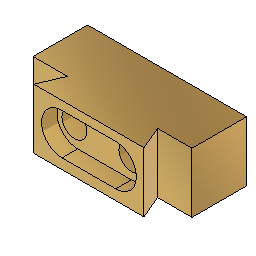
Low Profile Vice Base v5 (Autodesk Fusion 360 archive; units mm, degrees)
design "Vice Piece Hex Only"
Autodesk Fusion 360 part; units mm, degrees
sketch "Sketch1" plane through (0, 0, 0) normal (0, 0, 1) x (1, 0, 0)
  line L0 (-13.9084, 7.56) -> (36.9716, 7.56)
  line L1 (36.9716, 7.56) -> (36.9716, 25.03)
  line L2 (36.9716, 25.03) -> (-13.9084, 25.03)
  line L3 (-13.9084, 25.03) -> (-13.9084, 7.56)
  line L4 (-13.9084, 7.56) -> (-2.9084, 7.56) construction
  line L5 (36.9716, 7.56) -> (25.9716, 7.56) construction
  dimension "d4" = 50.88
  dimension "d5" = 17.47
  dimension "d7" = 11
  dimension "d8" = 11
  constraint horizontal L0
  constraint vertical L1
  constraint horizontal L2
  constraint vertical L3
  constraint perpendicular L3 L4
  constraint perpendicular L1 L5
  measures "d4" distance of L0.start L0.end
  measures "d5" distance of L0.start L2.end
  measures "d7" distance of L0.start L4.end
  measures "d8" distance of L0.end L5.end
sketch "Sketch2" plane through (0, 0, 0) normal (0, 0, 1) x (1, 0, 0)
  line L0 (11.5316, 0) -> (29.1316, 0)
  line L1 (11.5316, 0) -> (-6.0684, 0)
  line L2 (-13.9084, 7.56) -> (36.9716, 7.56)
  line L3 (-2.9084, 7.56) -> (-6.0684, 0)
  line L4 (25.9716, 7.56) -> (29.1316, 0)
  point P0 (-2.9084, 7.56)
  point P1 (25.9716, 7.56)
  dimension "d9" = 17.6
  dimension "d10" = 17.6
  dimension "d11" = 7.56
  constraint coincident P0 L3.start
  constraint coincident P1 L4.start
  measures "d9" distance of L0.start L0.end
  measures "d10" distance of L0.start L1.end
  measures "d11" distance of L0 L2
extrude "Extrude1" add sketch "Sketch1" sketch "Sketch2" along normal blind 19.16 of sketch 2
sketch "Sketch4" plane through (0, 0, 0) normal (0, 1, 0) x (1, 0, 0)
  circle A0 centre (2.9316, -9.8352) radius 6.57
  line L0 (-6.0684, 0) -> (-6.0684, -19.16)
  circle A1 centre (20.1316, -9.8352) radius 6.57
  line L1 (29.1316, 0) -> (29.1316, -19.16)
  line L2 (2.9316, -16.4052) -> (20.1316, -16.4052)
  line L3 (2.9387, -3.2652) -> (20.1316, -3.2652)
  dimension "d14" = 13.14
  dimension "d16" = 13.14
  dimension "d17" = 9
  dimension "d18" = 9
  constraint coincident A0 L2.start
  constraint coincident A1 L2.end
  constraint tangent A1 L2
  constraint coincident A0 L3.start
  constraint coincident A1 L3.end
  constraint tangent A1 L3
  measures "d14" diameter of A0
  measures "d16" diameter of A1
  measures "d17" distance of A1.centre L1
  measures "d18" distance of A0.centre L0
extrude "Extrude2" cut sketch "Sketch4" along normal blind 5
sketch "Sketch5" plane through (0, 25.03, 0) normal (0, 1, 0) x (-1, 0, 0)
  line L0 (-36.9716, 0) -> (13.9084, 0)
  line L1 (13.9084, 0) -> (13.9084, 19.16)
  line L2 (13.9084, 19.16) -> (-36.9716, 19.16)
  line L3 (-36.9716, 19.16) -> (-36.9716, 0)
  circle A0 centre (-20.1316, 9.58) radius 6.5
  circle A1 centre (-1.8809, 9.58) radius 6.5
  circle A2 centre (-20.1316, 9.58) radius 4
  circle A3 centre (-1.8809, 9.58) radius 4
  dimension "d21" = 13
  dimension "d22" = 13
  dimension "d24" = 9.58
  dimension "d25" = 9.58
  dimension "d26" = 8
  dimension "d27" = 8
  constraint concentric A0 A2
  constraint concentric A1 A3
  measures "d21" diameter of A0
  measures "d22" diameter of A1
  measures "d24" distance of L2 A1.centre
  measures "d25" distance of L2 A0.centre
  measures "d26" diameter of A2
  measures "d27" diameter of A3
extrude "Extrude3" cut sketch "Sketch5" against normal blind 5 contours A0 | A1
extrude "Extrude4" cut 2 faces at (2.6679, 25.03, 7.9458) (19.0151, 25.03, 9.0276) along direction (0, 1, 0) up to surface end surface through (0, 5, 0) normal (0, -1, 0) offset 0
equation "d12 = thickness"
equation "d19 = boltSink"
equation "d21 = boltH"
equation "d22 = boltH"
equation "thickness = 19.16 mm"
equation "d24 = ( 19.16 / 2 ) * 1 mm"
equation "d26 = bolt"
equation "d27 = bolt"
equation "d28 = -boltSink"
equation "boltH = 13 mm"
equation "boltSink = 5 mm"
equation "bolt = 8 mm"

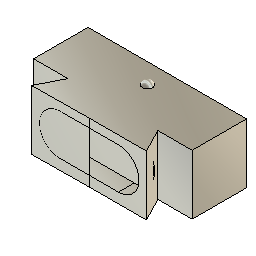
design "Vice Piece Base Body"
Autodesk Fusion 360 part; units mm, degrees
sketch "Sketch1" plane through (0, 0, 0) normal (0, 0, 1) x (1, 0, 0)
  line L0 (-13.9084, 7.56) -> (36.9716, 7.56)
  line L1 (36.9716, 7.56) -> (36.9716, 25.03)
  line L2 (36.9716, 25.03) -> (-13.9084, 25.03)
  line L3 (-13.9084, 25.03) -> (-13.9084, 7.56)
  line L4 (-13.9084, 7.56) -> (-2.9084, 7.56) construction
  line L5 (36.9716, 7.56) -> (25.9716, 7.56) construction
  dimension "d4" = 50.88
  dimension "d5" = 17.47
  dimension "d7" = 11
  dimension "d8" = 11
  constraint horizontal L0
  constraint vertical L1
  constraint horizontal L2
  constraint vertical L3
  constraint perpendicular L3 L4
  constraint perpendicular L1 L5
  measures "d4" distance of L0.start L0.end
  measures "d5" distance of L0.start L2.end
  measures "d7" distance of L0.start L4.end
  measures "d8" distance of L0.end L5.end
sketch "Sketch2" plane through (0, 0, 0) normal (0, 0, 1) x (1, 0, 0)
  line L0 (11.5316, 0) -> (29.8716, 0)
  line L1 (11.5316, 0) -> (-6.8074, -0.1898)
  line L2 (-13.9084, 7.56) -> (36.9716, 7.56)
  line L3 (-2.9084, 7.56) -> (-6.8074, -0.1898)
  line L4 (25.9716, 7.56) -> (29.8716, 0)
  point P0 (-2.9084, 7.56)
  point P1 (25.9716, 7.56)
  dimension "d9" = 18.34
  dimension "d10" = 18.34
  dimension "d11" = 7.56
  constraint coincident P0 L3.start
  constraint coincident P1 L4.start
  measures "d9" distance of L0.start L0.end
  measures "d10" distance of L0.start L1.end
  measures "d11" distance of L0 L2
extrude "Extrude1" add sketch "Sketch1" sketch "Sketch2" along normal blind 19.16 of sketch 2 makes body 1
sketch "Sketch4" plane through (0, 0, 0) normal (0, 1, 0) x (1, 0, 0)
  circle A0 centre (2.1926, -9.8352) radius 6.57
  line L0 (-6.8074, 0) -> (-6.8074, -19.16)
  circle A1 centre (20.8716, -9.8352) radius 6.57
  line L1 (29.8716, 0) -> (29.8716, -19.16)
  line L2 (2.1926, -16.4052) -> (20.8716, -16.4052)
  line L3 (2.1997, -3.2652) -> (20.8716, -3.2652)
  dimension "d14" = 13.14
  dimension "d16" = 13.14
  dimension "d17" = 9
  dimension "d18" = 9
  constraint coincident A0 L2.start
  constraint coincident A1 L2.end
  constraint tangent A1 L2
  constraint coincident A0 L3.start
  constraint coincident A1 L3.end
  constraint tangent A1 L3
  measures "d14" diameter of A0
  measures "d16" diameter of A1
  measures "d17" distance of A1.centre L1
  measures "d18" distance of A0.centre L0
extrude "Extrude2" cut sketch "Sketch4" along normal blind 5.08 bodies 1
sketch "Sketch5" plane through (0, 0, 19.16) normal (0, 0, 1) x (-1, 0, 0)
  line L0 (13.9084, -25.03) -> (13.9084, -7.56)
  line L1 (13.9084, -7.56) -> (2.9084, -7.56)
  line L2 (2.9084, -7.56) -> (6.8074, 0.1898)
  line L3 (6.8074, 0.1898) -> (-11.5316, 0)
  line L4 (-29.8716, 0) -> (-25.9716, -7.56)
  line L5 (-25.9716, -7.56) -> (-36.9716, -7.56)
  line L6 (-36.9716, -7.56) -> (-36.9716, -25.03)
  line L7 (-36.9716, -25.03) -> (13.9084, -25.03)
  circle A0 centre (-11.5316, -18.68) radius 1.75
  line L8 (-11.5316, 0) -> (-29.8716, 0)
  dimension "d21" = 3.5
  dimension "d22" = 6.35
  dimension "d23" = 25.44
  measures "d21" diameter of A0
  measures "d22" distance of L7 A0.centre
  measures "d23" distance of L0 A0.centre
sphere "SpherePrimitive1" add diameter 3.5 placed x (-1, 0, 0) y (0, -1, 0) z (0, 0, 1) at (11.5316, 18.68, 19.16) separate body makes body 2
move_body "MoveFace1" bodies 2 to x (1, 0, 0) y (0, 1, 0) z (0, 0, 1) at (0, 0, -0.5) on bodies 2
delete_face "DeleteFace1" 1 faces at (9.8725, 18.2663, 18.2876) on bodies 2
sphere "SpherePrimitive2" add diameter 3.5 placed x (-1, 0, 0) y (0, -1, 0) z (0, 0, 1) at (11.5316, 18.68, 19.16) separate body makes body 3
move_body "Move1" bodies 3 to x (1, 0, 0) y (0, 1, 0) z (0, 0, 1) at (0, 0, -0.5)
combine "Combine1" operation add target body 3 tool bodies 1
equation "d9 = 17.6 mm + 0.74 mm"
equation "d10 = 17.6 mm + 0.74 mm"
equation "d23 = ( 50.88 / 2 ) * 1 mm"
